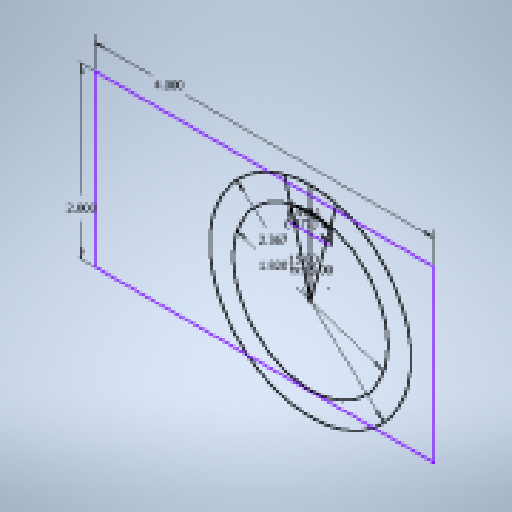
# Autodesk Inventor part: Part141
Saved by Autodesk Inventor 2023 (Build 270158000, 158)
## iProperties
Created: 2023-03-28
Part Number: Part141
Material: Generic
Document SubType Name: Modeling
Designer: Gabriel - T3 CAD
Density: 1 g/cm^3
Appearance: Default
Author: Gabriel - T3 CAD
Autodesk Inventor part; units mm, degrees
ref_plane "YZ Plane" through (0, 0, 0) normal (1, 0, 0) x (0, 1, 0)
ref_plane "XZ Plane" through (0, 0, 0) normal (0, 1, 0) x (-1, 0, 0)
ref_plane "XY Plane" through (0, 0, 0) normal (0, 0, 1) x (1, 0, 0)
sketch "Sketch2" plane through (0, 0, 0) normal (0, 0, 1) x (1, 0, 0)
  circle A0 centre (0, 0) radius 23.114
  circle A1 centre (0, 0) radius 5.969
  line L0 (-23.114, 5.969) -> (23.114, 5.969)
  line L1 (23.114, 5.969) -> (23.114, -5.969)
  line L2 (23.114, -5.969) -> (-23.114, -5.969)
  line L3 (-23.114, -5.969) -> (-23.114, 5.969)
  line L4 (29.464, -12.319) -> (-29.464, -12.319)
  line L5 (-29.464, -12.319) -> (-29.464, 12.319)
  line L6 (-29.464, 12.319) -> (29.464, 12.319)
  line L7 (29.464, 12.319) -> (29.464, -12.319)
  line L8 (29.464, -12.319) -> (-29.464, 12.319) construction
  line L9 (-29.464, -12.319) -> (29.464, 12.319) construction
  line L10 (23.114, 5.969) -> (23.114, -5.969)
  line L11 (23.114, -5.969) -> (29.464, -5.969)
  line L12 (29.464, -5.969) -> (29.464, 5.969)
  line L13 (29.464, 5.969) -> (23.114, 5.969)
  dimension "d14" = 46.228
  dimension "d15" = 11.938
  dimension "d16" = 46.228
  dimension "d17" = 11.938
  dimension "d18" = 23.114
  dimension "d19" = 5.969
  dimension "d20" = 24.638
  dimension "d21" = 58.928
  constraints: 28 end point, 6 parallel, 3 perpendicular, 2 centre point, 2 coincident, 2 horizontal, 2 midpoint
  measures "d14" diameter of A0
  measures "d15" diameter of A1
  measures "d16" distance of L1.end L2.end
  measures "d17" distance of L0.end L1.end
  measures "d18" distance from line of point (0, 0) L1
  measures "d19" distance from line of point (0, 0) L2
  measures "d20" distance of L4.end L5.end
  measures "d21" distance of L5.end L6.end
extrude "Extrusion2" add sketch "Sketch2" along normal blind 7.95 contours L0 A0 L6 | A0 L6 L7 L13 L0 | L2 L11 L7 L4 A0 | A0 L4 L2 | A0 L0 L3 L2 L4 L5 L6
extrude "Extrusion3" add sketch "Sketch2" against normal blind 6.35 contours A0 L2 A1 L0 | L1 L2 A0 | A0 L0 L1 | L1 L13 L7 L11 | L0 A0 L6 | A0 L6 L7 L13 L0 | L2 L11 L7 L4 A0 | A0 L4 L2 | A1 | A1 L2 A0 L0 | A0 L0 L3 L2 L4 L5 L6 | A0 L3 L0 | L2 L3 A0
ref_plane "Work Plane1" through (0, 0, 25.85) normal (0, 0, 1) x (1, 0, 0)
equation "\"d18\" = 0.5 * d16"
equation "\"d19\" = 0.5 * d17"
body "Solid2"
